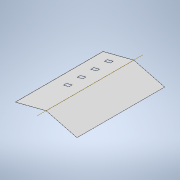
# Autodesk Inventor part: garageRoof
Saved by Autodesk Inventor 2022.1 (Build 261234000, 234)
## iProperties
Created: 2021-07-13
Part Number: garageRoof
Material: Generic
Document SubType Name: Modeling
Designer: robst
Density: 1 g/cm^3
Appearance: Default
Author: robst
Autodesk Inventor part; units mm, degrees
ref_plane "YZ Plane" through (0, 0, 0) normal (1, 0, 0) x (0, 1, 0)
ref_plane "XY Plane" through (0, 0, 0) normal (0, 0, 1) x (1, 0, 0)
ref_plane "southPlaneOfRoof" through (0, 0, 0) normal (-0.2492815, 0.9684311, 0) x (0, 0, 1)
ref_plane "norhtPlaneOfRoof" through (0, 0, 0) normal (0.2492815, 0.9684311, 0) x (0, 0, 1)
sketch "Sketch3" plane through (0, 0, 0) normal (-0.2492815, 0.9684311, 0) x (0, 0, 1)
  line L0 (0, 0) -> (-19507.2, 0)
  line L1 (-19507.2, 0) -> (-19507.2, -7086.6)
  line L2 (0, 0) -> (0, -7086.6)
  line L3 (0, -7086.6) -> (0, -25.4)
  line L4 (-19507.2, -7086.6) -> (0, -7086.6)
  line L5 (-17703.8, -4203.7) -> (-17043.4, -4203.7)
  line L6 (-17043.4, -4203.7) -> (-17043.4, -2908.3)
  line L7 (-17043.4, -2908.3) -> (-17703.8, -2908.3)
  line L8 (-17703.8, -2908.3) -> (-17703.8, -4203.7)
  line L9 (-14655.8, -4191) -> (-13995.4, -4191)
  line L10 (-13995.4, -4191) -> (-13995.4, -2895.6)
  line L11 (-13995.4, -2895.6) -> (-14655.8, -2895.6)
  line L12 (-14655.8, -2895.6) -> (-14655.8, -4191)
  line L13 (-11620.5, -4165.6) -> (-10960.1, -4165.6)
  line L14 (-10960.1, -4165.6) -> (-10960.1, -2870.2)
  line L15 (-10960.1, -2870.2) -> (-11620.5, -2870.2)
  line L16 (-11620.5, -2870.2) -> (-11620.5, -4165.6)
  line L17 (-8572.5, -4191) -> (-7912.1, -4191)
  line L18 (-7912.1, -4191) -> (-7912.1, -2895.6)
  line L19 (-7912.1, -2895.6) -> (-8572.5, -2895.6)
  line L20 (-8572.5, -2895.6) -> (-8572.5, -4191)
  dimension "d9" = 19507.2
  dimension "d10" = 7086.6
  dimension "d11" = 7061.2
  dimension "d15" = 660.4
  dimension "d16" = 1295.4
  dimension "d17" = 1803.4
  dimension "d18" = 2387.6
  dimension "d19" = 2374.9
  dimension "d20" = 2387.6
  dimension "d21" = 2908.3
  dimension "d22" = 2895.6
  dimension "d23" = 2870.2
  dimension "d24" = 2895.6
  constraints: 42 end point, 14 parallel, 6 horizontal, 4 perpendicular, 2 vertical, 1 point on line
  measures "d9" distance of L0.start L0.end
  measures "d10" distance of L0.end L1.end
  measures "d11" distance of L2.end L3.end
  measures "d15" distance of L5.start L5.end
  measures "d16" distance of L7.end L5.start
  measures "d17" distance between parallel lines of L8 L1
  measures "d18" distance between parallel lines of L12 L6
  measures "d19" distance between parallel lines of L16 L10
  measures "d20" distance between parallel lines of L20 L14
  measures "d21" distance between parallel lines of L7 L0
  measures "d22" distance between parallel lines of L11 L0
  measures "d23" distance between parallel lines of L15 L0
  measures "d24" distance between parallel lines of L19 L0
sketch "Sketch4" plane through (0, 0, 0) normal (0.2492815, 0.9684311, 0) x (0, 0, 1)
  line L0 (0, 0) -> (0, 7086.6)
  line L1 (0, 0) -> (-19507.2, 0)
  line L2 (-19507.2, 0) -> (-19507.2, 7086.6)
  line L3 (-19507.2, 7086.6) -> (0, 7086.6)
  dimension "d12" = 7086.6
  dimension "d13" = 19507.2
  dimension "d14" = 7086.6
  constraints: 8 end point, 1 horizontal, 1 perpendicular, 1 vertical
  measures "d12" distance of L0.start L0.end
  measures "d13" distance of L0.start L1.end
  measures "d14" distance of L1.end L2.end
extrude "Extrusion2" add sketch "Sketch3" against normal blind 25.4
extrude "Extrusion3" add sketch "Sketch4" against normal blind 25.4
equation "\"pitch_4_12\" = 14.435deg"
equation "\"d7\" = pitch_4_12"
equation "\"d8\" = -pitch_4_12"
body "Solid2"
